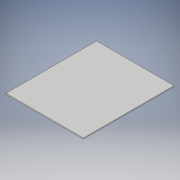
# Autodesk Inventor part: BrainBoxTopBot
Saved by Autodesk Inventor 2018 (Build 220112000, 112)
## iProperties
Created: 2019-01-10
Part Number: BrainBoxTopBot
Material: Generic
Document SubType Name: Modeling
Designer: snipe
Density: 1 g/cm^3
Appearance: Default
Author: snipe
Autodesk Inventor part; units mm, degrees
ref_plane "YZ Plane" through (0, 0, 0) normal (1, 0, 0) x (0, 1, 0)
ref_plane "XZ Plane" through (0, 0, 0) normal (0, 1, 0) x (-1, 0, 0)
ref_plane "XY Plane" through (0, 0, 0) normal (0, 0, 1) x (1, 0, 0)
sketch "Sketch1" plane through (0, 0, 0) normal (0, 1, 0) x (-1, 0, 0)
  line L0 (0, -208.026) -> (0, 208.026) projected
  line L1 (-177.8, 0) -> (177.8, 0) projected
  line L2 (177.8, 0) -> (-177.8, 0) projected
  line L3 (0, -208.026) -> (0, 208.026) projected
  line L4 (127, 148.59) -> (-127, 148.59)
  line L5 (-127, 148.59) -> (-127, -148.59)
  line L6 (-127, -148.59) -> (127, -148.59)
  line L7 (127, -148.59) -> (127, 148.59)
  line L8 (127, 148.59) -> (-127, -148.59) construction
  line L9 (-127, 148.59) -> (127, -148.59) construction
  point P0 (0, 0)
  dimension "d0" = 254
  dimension "d1" = 297.18
  constraints: 12 end point, 2 midpoint, 2 parallel, 1 horizontal, 1 perpendicular
  measures "d0" distance of L6.end L5.end
  measures "d1" distance of L5.end L4.end
extrude "Extrusion1" add sketch "Sketch1" along normal mid plane 3.175
body "Solid1"
